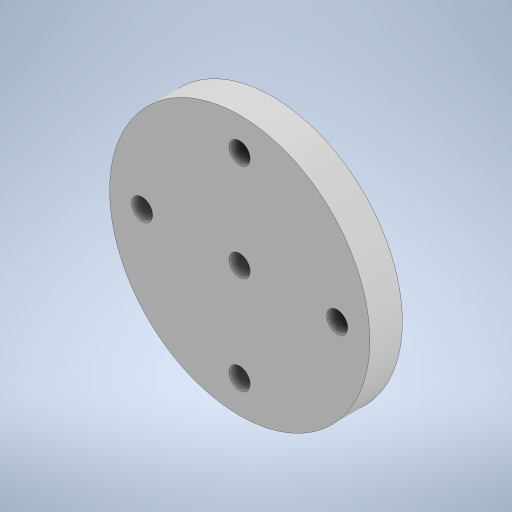
# Autodesk Inventor part: gearbox_connector1
Saved by Autodesk Inventor 2023 (Build 270158000, 158)
## iProperties
Created: 2023-05-28
Part Number: gearbox_connector1
Material: 一般
Document SubType Name: Modeling
Designer: 310611102
Density: 1 g/cm^3
Appearance: 預設
Author: 310611102
Autodesk Inventor part; units mm, degrees
ref_plane "YZ Plane" through (0, 0, 0) normal (1, 0, 0) x (0, 1, 0)
ref_plane "XZ Plane" through (0, 0, 0) normal (0, 1, 0) x (-1, 0, 0)
ref_plane "XY Plane" through (0, 0, 0) normal (0, 0, 1) x (1, 0, 0)
sketch "Sketch1" plane through (0, 0, 0) normal (0, 0, 1) x (1, 0, 0)
  circle A0 centre (0, 0) radius 20
  circle A1 centre (0, 0) radius 1.6
  circle A2 centre (0, 15) radius 1.6
  circle A3 centre (-15, 0) radius 1.6
  circle A4 centre (0, -15) radius 1.6
  circle A5 centre (15, 0) radius 1.6
  dimension "d0" = 40
  dimension "d9" = 3.2
  dimension "d10" = 3.2
  dimension "d13" = 360
  dimension "d15" = 30
  constraints: 6 centre point, 2 coincident, 1 vertical alignment, 9 other
  measures "d0" diameter of A0
  measures "d9" diameter of A1
  measures "d10" diameter of A2
  measures "d15" distance of A4.centre A2.centre
extrude "Extrusion1" add sketch "Sketch1" along normal blind 5
body "Solid1"
